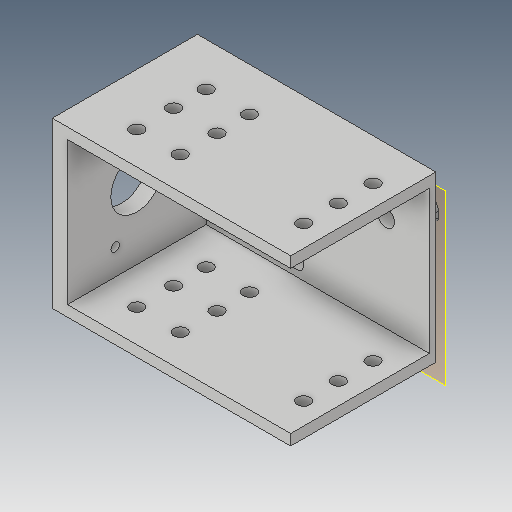
# Autodesk Inventor part: 10_Adapterplate_Laser
Saved by Autodesk Inventor 2019 (Build 230136000, 136)
## iProperties
Created: 2019-04-21
Part Number: 10_Adapterplate_Laser
Material: Generic
Document SubType Name: Modeling
Designer: diederichbenedict
Density: 1 g/cm^3
Appearance: Default
Author: diederichbenedict
Autodesk Inventor part; units mm, degrees
ref_plane "YZ Plane" through (0, 0, 0) normal (1, 0, 0) x (0, 1, 0)
ref_plane "Work Plane1" through (0, 0, 0) normal (0, 0, 1) x (1, 0, 0)
ref_plane "Work Plane2" through (-26.5718, -7.4484, 7) normal (0, 0, -1) x (0, 1, 0)
sketch "Sketch1" plane through (0, 0, 0) normal (0, 0, 1) x (1, 0, 0)
  line L0 (-10.7718, 17.6016) -> (-13.2718, 17.6016) construction
  line L1 (-13.2718, 10.7516) -> (-13.2718, 17.6016)
  line L2 (-12.2718, 10.7516) -> (-13.2718, 10.7516) construction
  line L3 (-12.2718, -9.2484) -> (-12.2718, 10.7516) construction
  line L4 (-13.2718, -9.2484) -> (-12.2718, -9.2484) construction
  line L5 (-13.2718, 9.2516) -> (-13.2718, -9.2484) construction
  line L6 (-17.2718, 9.2516) -> (-13.2718, 9.2516) construction
  line L7 (-17.2718, 8.5516) -> (-17.2718, 9.2516) construction
  line L8 (-16.7718, 8.5516) -> (-17.2718, 8.5516) construction
  line L9 (-16.7718, -6.8984) -> (-16.7718, 8.5516) construction
  line L10 (-15.5718, -6.8984) -> (-16.7718, -6.8984) construction
  line L11 (-15.5718, -10.1675) -> (-15.5718, -6.8984) construction
  line L12 (-15.5718, -10.1675) -> (-15.0718, -10.1675) construction
  arc A0 (-11.4718, -11.3675) -> (-15.0718, -10.1675) centre (-13.4718, -11.3675) ccw construction
  line L13 (-11.4718, -11.3675) -> (-11.4718, -15.0734) construction
  arc A1 (-11.4718, -15.0734) -> (0.1282, -17.7415) centre (-0.4485, 6.3019) ccw construction
  line L14 (0.1282, -17.7415) -> (0.1282, -16.3415) construction
  line L15 (0.1282, -16.3415) -> (-1.8718, -16.3415) construction
  line L16 (-1.8718, -16.3415) -> (-2.3718, -15.8415) construction
  line L17 (-2.3718, -15.8415) -> (-4.3718, -15.8415) construction
  line L18 (-4.3718, -15.8415) -> (-4.8718, -15.3415) construction
  line L19 (-4.8718, -15.3415) -> (-6.8718, -15.3415) construction
  line L20 (-6.8718, -15.3415) -> (-10.4718, -11.7415) construction
  line L21 (-10.4718, -11.7415) -> (-10.4718, -8.9915) construction
  arc A2 (-8.1012, -8.7277) -> (-10.4718, -8.9915) centre (-9.3012, -8.7277) ccw construction
  line L22 (-8.1012, -8.7277) -> (-8.1012, -7.7277) construction
  line L23 (-8.1012, -7.7277) -> (-3.5718, -3.1984) construction
  line L24 (-3.5718, -3.1984) -> (12.4282, -3.1984) construction
  line L25 (12.4282, 10.2016) -> (12.4282, -3.1984)
  arc A3 (14.4282, 12.2016) -> (12.4282, 10.2016) centre (14.4282, 10.2016) ccw
  line L26 (15.5282, 12.2016) -> (14.4282, 12.2016)
  arc A4 (15.5282, 12.2016) -> (16.5282, 13.2016) centre (15.5282, 13.2016) ccw
  line L27 (16.5282, 14.5766) -> (16.5282, 13.2016)
  arc A5 (16.5282, 14.5766) -> (14.5282, 16.5766) centre (14.5282, 14.5766) ccw
  line L28 (14.5282, 16.5766) -> (-8.9532, 16.5766)
  arc A6 (-10.7718, 17.6016) -> (-9.296, 16.5766) centre (-10.7718, 16.0266) ccw construction
  line L29 (0.7782, 12.3516) -> (5.1782, 12.3516) construction
  line L30 (5.1782, 12.3516) -> (5.1782, 1.1016) construction
  line L31 (5.1782, 1.1016) -> (0.7782, 1.1016) construction
  line L32 (0.7782, 1.1016) -> (0.7782, 0.0766) construction
  line L33 (0.7782, 0.0766) -> (-3.4218, 0.0766) construction
  line L34 (-3.4218, 0.0766) -> (-3.4218, 1.1016) construction
  line L35 (-3.4218, 1.1016) -> (-7.8218, 1.1016) construction
  line L36 (-7.8218, 1.1016) -> (-7.8218, 12.3516) construction
  line L37 (-7.8218, 12.3516) -> (-3.4218, 12.3516) construction
  line L38 (-3.4218, 12.3516) -> (-3.4218, 13.3766) construction
  line L39 (-3.4218, 13.3766) -> (0.7782, 13.3766) construction
  line L40 (0.7782, 13.3766) -> (0.7782, 12.3516) construction
  circle A7 centre (11.3782, 14.2016) radius 1.575 construction
  circle A8 centre (-9.3012, -4.7277) radius 1.575 construction
  circle A9 centre (14.3782, 14.2016) radius 0.75 construction
  circle A10 centre (11.3782, 14.2016) radius 2
  arc A11 (-11.8345, 17.6016) -> (-8.9532, 16.5766) centre (-10.7718, 16.0266) ccw
  circle A12 centre (-9.3012, -4.7277) radius 1.8
  line L41 (-8.9532, 16.5766) -> (14.5282, 16.5766)
  line L42 (12.4282, 10.2016) -> (12.4282, -3.1984)
  line L43 (12.4282, -3.1984) -> (-3.5718, -3.1984)
  line L44 (-3.5718, -3.1984) -> (-8.1012, -7.7277)
  line L45 (-8.1012, -7.7277) -> (-12.2718, -7.7277)
  line L46 (-12.2718, -7.7277) -> (-12.2718, 10.7516)
  line L47 (-13.2718, 10.7516) -> (-12.2718, 10.7516)
  line L48 (-13.2718, 10.7516) -> (-13.2718, 17.6016)
  line L49 (-13.2718, 17.6016) -> (-11.8345, 17.6016)
  arc A13 (14.4282, 12.2016) -> (12.4282, 10.2016) centre (14.4282, 10.2016) ccw
  arc A14 (16.5282, 14.5766) -> (14.5282, 16.5766) centre (14.5282, 14.5766) ccw
  arc A15 (15.5282, 12.2016) -> (16.5282, 13.2016) centre (15.5282, 13.2016) ccw
  line L50 (16.5282, 14.5766) -> (16.5282, 13.2016)
  line L51 (15.5282, 12.2016) -> (14.4282, 12.2016)
  line L52 (12.4282, 10.2016) -> (12.4282, -3.1984) projected
  arc A16 (14.4282, 12.2016) -> (12.4282, 10.2016) centre (14.4282, 10.2016) ccw projected
  line L53 (15.5282, 12.2016) -> (14.4282, 12.2016) projected
  arc A17 (15.5282, 12.2016) -> (16.5282, 13.2016) centre (15.5282, 13.2016) ccw projected
  line L54 (16.5282, 14.5766) -> (16.5282, 13.2016) projected
  arc A18 (16.5282, 14.5766) -> (14.5282, 16.5766) centre (14.5282, 14.5766) ccw projected
  line L55 (-12.2718, -6.8984) -> (-7.2718, -6.8984)
  line L56 (-13.2718, 10.7516) -> (-13.2718, 17.6016) projected
  line L57 (14.5282, 16.5766) -> (-9.296, 16.5766) projected
  point P0 (0, 0)
  dimension "d0" = 4
  dimension "d1" = 3.8
  dimension "d2" = 3.6
  constraints: 34 end point, 16 point on circle, 9 centre point, 5 point on line, 4 collinear, 4 perpendicular, 3 coincident, 2 concentric, 2 tangent
  measures "d0" diameter of A10
  measures "d1" diameter of A11
  measures "d2" diameter of A12
extrude "Extrusion1" add sketch "Sketch1" along normal up to surface (7 mm away) contours L1 L49 A11 L28 A5 L27 A4 L26 A3 L25 L43 L44 L55 L46 L47
sketch "Sketch3" plane through (0, 0, 7) normal (0, 0, 1) x (1, 0, 0)
  circle A0 centre (-10.7718, 16.0266) radius 1.575 projected
  arc A1 (-8.9532, 16.5766) -> (-11.8345, 17.6016) centre (-10.7718, 16.0266) ccw projected
  circle A2 centre (-10.7718, 16.0266) radius 1.9
  line L0 (-15.2532, -9.3857) -> (-5.307, -9.3857)
  line L1 (-5.307, -9.3857) -> (-5.307, -6.9163)
  line L2 (-5.307, -6.9163) -> (-15.2532, -6.9163)
  line L3 (-15.2532, -6.9163) -> (-15.2532, -9.3857)
  point P0 (0, 0)
  constraints: 8 end point, 2 parallel, 1 coincident, 1 horizontal, 1 perpendicular, 3 other
extrude "Extrusion3" cut sketch "Sketch3" against normal through all contours A0 | A2 A1 | L3 L2 L1 L0
sketch "Sketch4" plane through (-3.5718, -3.1984, 7) normal (0, 0, 1) x (1, 0, 0)
  circle A0 centre (-8, 19.25) radius 1 construction
  circle A1 centre (-8, 11.75) radius 1 construction
  circle A2 centre (-18, 19.25) radius 1 construction
  circle A3 centre (20, 3.75) radius 1 construction
  circle A4 centre (20, 11.75) radius 1 construction
  circle A5 centre (20, 19.75) radius 1 construction
  circle A6 centre (-18, 11.75) radius 1 construction
  circle A7 centre (-18, 3.25) radius 1 construction
  circle A8 centre (-8, 3.25) radius 1.0474 construction
  line L0 (25, 27.75) -> (25, -4.25) construction
  line L1 (25, 27.75) -> (-23, 27.75) construction
  line L2 (-23, -4.25) -> (-23, 27.75) construction
  line L3 (25, -4.25) -> (-23, -4.25) construction
  line L4 (25, -7.25) -> (-30, -7.25)
  line L5 (-30, -7.25) -> (-30, 30.75)
  line L6 (-30, 30.75) -> (25, 30.75)
  line L7 (25, 30.75) -> (25, -7.25)
  line L8 (-30, -16.9963) -> (-30, 50.9756)
  circle A9 centre (-5.7293, -1.5293) radius 1.8 projected
  circle A10 centre (14.95, 17.4) radius 2 projected
  arc A11 (-8.2627, 20.8) -> (-5.3813, 19.775) centre (-7.2, 19.225) ccw projected
  arc A12 (-8.2627, 20.8) -> (-5.3813, 19.775) centre (-7.2, 19.225) ccw projected
  line L9 (-8.2627, 20.8) -> (-9.7, 20.8) projected
  line L10 (-9.7, 20.8) -> (-9.7, 13.95) projected
  line L11 (-9.7, 13.95) -> (-8.7, 13.95) projected
  line L12 (-8.7, 13.95) -> (-8.7, -3.7) projected
  line L13 (-3.7, -3.7) -> (0, 0) projected
  line L14 (0, 0) -> (16, 0) projected
  line L15 (16, 0) -> (16, 13.4) projected
  arc A13 (18, 15.4) -> (16, 13.4) centre (18, 13.4) ccw projected
  line L16 (18, 15.4) -> (19.1, 15.4) projected
  arc A14 (19.1, 15.4) -> (20.1, 16.4) centre (19.1, 16.4) ccw projected
  line L17 (20.1, 16.4) -> (20.1, 17.775) projected
  arc A15 (20.1, 17.775) -> (18.1, 19.775) centre (18.1, 17.775) ccw projected
  line L18 (18.1, 19.775) -> (-5.3813, 19.775) projected
  circle A16 centre (-5.7293, -1.5293) radius 1.8 projected
  circle A17 centre (14.95, 17.4) radius 2 projected
  line L19 (-8.7, -3.7) -> (-3.7, -3.7) projected
  line L20 (18.1, 19.775) -> (-5.3813, 19.775) projected
  circle A18 centre (-7.2, 19.225) radius 1.9
  point P0 (3.5718, 3.1984)
  point P1 (-30, 11.75)
  dimension "d10" = 3
  dimension "d11" = 3
  dimension "d12" = 0
  constraints: 10 end point, 2 parallel, 1 coincident, 1 horizontal, 1 midpoint, 1 perpendicular, 1 point on line, 1 vertical, 5 other
  measures "d10" distance between parallel lines of L4 L3
  measures "d11" distance between parallel lines of L6 L1
  measures "d12" distance between parallel lines of L0 L7
extrude "Extrusion4" add sketch "Sketch4" against normal blind 1.5 contours L4 L5 L6 L7 | A11 L18 A15 L17 A14 L16 A13 L15 L14 L13 L19 L12 L11 L10 L9
sketch "Sketch5" plane through (-33.5718, -10.4484, 7) normal (0, 0, 1) x (1, 0, 0)
  line L0 (55, 0) -> (0, 0) projected
  line L1 (55, 38) -> (55, 0) projected
  line L2 (0, 38) -> (55, 38) projected
  line L3 (0, 0) -> (0, 38) projected
  circle A0 centre (22, 26.5) radius 1 construction
  circle A1 centre (22, 19) radius 1 construction
  circle A2 centre (12, 26.5) radius 1 construction
  circle A3 centre (50, 11) radius 1 construction
  circle A4 centre (50, 19) radius 1 construction
  circle A5 centre (50, 27) radius 1 construction
  circle A6 centre (12, 19) radius 1 construction
  circle A7 centre (12, 10.5) radius 1 construction
  circle A8 centre (22, 10.5) radius 1.0474 construction
  line L4 (55, 35) -> (55, 3) construction
  line L5 (55, 35) -> (7, 35) construction
  line L6 (7, 3) -> (7, 35) construction
  line L7 (55, 3) -> (7, 3) construction
  line L8 (55, 38) -> (55, 0) projected
  line L9 (0, 0) -> (0, 38) projected
  line L10 (55, 0) -> (0, 0)
  line L11 (0, 0) -> (0, 2.5)
  line L12 (0, 2.5) -> (55, 2.5)
  line L13 (55, 2.5) -> (55, 0)
  line L14 (0, 38) -> (55, 38) projected
  line L15 (55, 38) -> (0, 38)
  line L16 (0, 38) -> (0, 35.5)
  line L17 (0, 35.5) -> (55, 35.5)
  line L18 (55, 35.5) -> (55, 38)
  line L19 (0, 2.5) -> (3.5, 2.5)
  line L20 (3.5, 2.5) -> (3.5, 35.5)
  line L21 (3.5, 35.5) -> (0, 35.5)
  line L22 (0, 35.5) -> (0, 2.5)
  point P0 (33.5718, 10.4484)
  dimension "d15" = 2.5
  dimension "d16" = 2.5
  dimension "d17" = 3.5
  constraints: 24 end point, 6 parallel, 3 horizontal, 3 perpendicular, 3 point on line
  measures "d15" distance of L10.end L11.end
  measures "d16" distance of L16.end L15.end
  measures "d17" distance of L21.end L20.end
ref_plane "Work Plane3" through (-26.5718, -7.4484, 39) normal (0, 0, 1) x (1, 0, 0)
extrude "Extrusion5" add sketch "Sketch5" along normal up to surface (32 mm away) contours L0 L3 L12 L1 | L3 L17 L20 L12 | L17 L3 L2 L1
sketch "Sketch6" plane through (-33.5718, 27.5516, 5.5) normal (0, 1, 0) x (1, 0, 0)
  circle A0 centre (22, -10) radius 1 projected
  circle A1 centre (22, -17.5) radius 1 projected
  circle A2 centre (12, -10) radius 1 projected
  circle A3 centre (50, -25.5) radius 1 projected
  circle A4 centre (50, -17.5) radius 1 projected
  circle A5 centre (50, -9.5) radius 1 projected
  circle A6 centre (12, -17.5) radius 1 projected
  circle A7 centre (12, -26) radius 1 projected
  circle A8 centre (22, -26) radius 1.0474 projected
  line L0 (55, -1.5) -> (55, -33.5) projected
  line L1 (55, -1.5) -> (7, -1.5) projected
  line L2 (7, -33.5) -> (7, -1.5) projected
  line L3 (55, -33.5) -> (7, -33.5) projected
  point P0 (33.5718, 5.5)
hole "Hole1" at (16.4282, 27.5516, 31) at (16.4282, 27.5516, 23) at (16.4282, 27.5516, 15) at (-11.5718, 27.5516, 31.5) at (-21.5718, 27.5516, 31.5) at (-11.5718, 27.5516, 23) at (-11.5718, 27.5516, 15.5) at (-21.5718, 27.5516, 15.5) at (-21.5718, 27.5516, 23) direction (0, -1, 0) diameter 3 end through all
sketch "Sketch7" plane through (-33.5718, -10.4484, 5.5) normal (-1, 0, 0) x (0, 0, 1)
  circle A0 centre (17.5, 19) radius 6 projected
  circle A1 centre (22.5, 8.5) radius 1 projected
  circle A2 centre (7, 30) radius 1 projected
  circle A3 centre (27.5, 36.5) radius 1 projected
  point P0 (-5.5, 10.4484)
extrude "Extrusion6" cut sketch "Sketch7" against normal blind 15
sketch "Sketch8" plane through (21.4282, -7.9484, 7) normal (0, 0, 1) x (1, 0, 0)
  line L0 (-27.5, 18.3) -> (-18, 18.3) projected
  line L1 (-27.5, 11.05) -> (-27.5, 18.3) projected
  line L2 (-18, 11.05) -> (-27.5, 11.05) projected
  line L3 (-18, 18.3) -> (-18, 11.05) projected
  circle A0 centre (-27.7, 7.025) radius 0.45 projected
  circle A1 centre (-17.75, 22.325) radius 0.45 projected
  line L4 (-18.95, 22.325) -> (-18.95, 20.825) projected
  arc A2 (-16.55, 22.325) -> (-18.95, 22.325) centre (-17.75, 22.325) ccw projected
  line L5 (-16.55, 20.825) -> (-16.55, 22.325) projected
  line L6 (-15.8, 20.825) -> (-16.55, 20.825) projected
  line L7 (-15.8, 8.525) -> (-15.8, 20.825) projected
  line L8 (-19.35, 8.525) -> (-15.8, 8.525) projected
  line L9 (-25.35, 8.525) -> (-19.35, 8.525) projected
  line L10 (-26.5, 8.525) -> (-25.35, 8.525) projected
  line L11 (-26.5, 7.025) -> (-26.5, 8.525) projected
  arc A3 (-28.9, 7.025) -> (-26.5, 7.025) centre (-27.7, 7.025) ccw projected
  line L12 (-28.9, 8.525) -> (-28.9, 7.025) projected
  line L13 (-29.7, 8.525) -> (-28.9, 8.525) projected
  line L14 (-29.7, 20.825) -> (-29.7, 8.525) projected
  line L15 (-25.35, 20.825) -> (-29.7, 20.825) projected
  line L16 (-19.35, 20.825) -> (-25.35, 20.825) projected
  line L17 (-18.95, 20.825) -> (-19.35, 20.825) projected
  circle A4 centre (-23.875, 14.675) radius 3.625
  circle A5 centre (-22.75, 14.675) radius 3.625
  circle A6 centre (-23.3021, 14.675) radius 3.625
  point P0 (-21.4282, 7.9484)
  constraints: 5 tangent, 3 centre point
hole "Hole2" at (-2.4468, 6.7266, 7) direction (0, 0, -1) diameter 3.6 end through all counterbore diameter 7 counterbore depth 3
body "Solid1"
